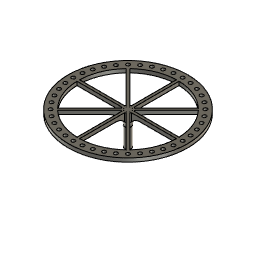
Reaction_Wheel (Autodesk Fusion 360 design; units mm, degrees)
Autodesk Fusion 360 part; units mm, degrees
note: some values were not read from the file. Chosen so that the rebuilt part matches the saved one: which pieces of a blend or face edit are solid.
sketch "스케치1" plane through (0, 0, 0) normal (0, 0, 1) x (1, 0, 0)
  circle A0 centre (0, 0) radius 1.6
  circle A1 centre (0, 0) radius 3.3
  dimension "d1" = 3.2
  dimension "d2" = 6.6
  constraint coincident A0.centre A1.centre
  measures "d1" diameter of A0
  measures "d2" diameter of A1
extrude "돌출1" add sketch "스케치1" along normal blind 30 makes body 1
sketch "스케치2" plane through (0, 0, 30) normal (0, 0, 1) x (-1, 0, 0)
  circle A0 centre (0, 0) radius 60
  circle A1 centre (0, 0) radius 50
  circle A2 centre (0, 0) radius 3.3
  line L0 (1.310929, -3.028443) -> (1.310929, -49.982812)
  line L1 (-1.310929, -3.028443) -> (-1.310929, -49.982812)
  line L2 (3.068399, -1.214465) -> (36.270152, -34.416218)
  line L3 (1.214465, -3.068399) -> (34.416218, -36.270152)
  line L4 (3.028443, 1.310929) -> (49.982812, 1.310929)
  line L5 (3.028443, -1.310929) -> (49.982812, -1.310929)
  line L6 (1.214465, 3.068399) -> (34.416218, 36.270152)
  line L7 (3.068399, 1.214465) -> (36.270152, 34.416218)
  line L8 (-1.310929, 3.028443) -> (-1.310929, 49.982812)
  line L9 (1.310929, 3.028443) -> (1.310929, 49.982812)
  line L10 (-3.068399, 1.214465) -> (-36.270152, 34.416218)
  line L11 (-1.214465, 3.068399) -> (-34.416218, 36.270152)
  line L12 (-3.028443, -1.310929) -> (-49.982812, -1.310929)
  line L13 (-3.028443, 1.310929) -> (-49.982812, 1.310929)
  line L14 (-1.214465, -3.068399) -> (-34.416218, -36.270152)
  line L15 (-3.068399, -1.214465) -> (-36.270152, -34.416218)
  circle A3 centre (0, 0) radius 5
  dimension "d5" = 120
  dimension "d11" = 100
  dimension "d13" = 360
  dimension "d21" = 10
  constraint coincident A0.centre A1.centre
  constraint concentric A1 A3
  measures "d5" diameter of A0
  measures "d11" diameter of A1
  measures "d21" diameter of A3
extrude "돌출3" add sketch "스케치2" along normal blind 2.7 separate body contours A0 | A1 L4 L5 A3 | A1 L6 L7 A3 | A2 L2 L4 L5 L7 A3 | L4 L7 A3 | A1 L2 L3 A3 | L2 L5 A3 | A2 L4 L6 L7 L9 A3 | A2 L0 L2 L3 L5 A3 | A1 L8 L9 A3 | L6 L9 A3 | A2 | A1 L0 L1 A3 | L0 L3 A3 | A2 L6 L8 L9 L11 A3 | A2 L0 L1 L3 L14 A3 | A1 L10 L11 A3 | L8 L11 A3 | A1 L14 L15 A3 | L1 L14 A3 | A2 L8 L10 L11 L13 A3 | A2 L1 L12 L14 L15 A3 | A1 L12 L13 A3 | L10 L13 A3 | L12 L15 A3 | A2 L10 L12 L13 L15 A3 picked at (-0.145674, 56.554182) picked at (19.987758, -0.584166) picked at (24.747837, 24.747837) picked at (3.728779, 1.147432) picked at (4.131776, 1.711438) picked at (24.747837, -24.747837) picked at (4.131776, -1.711438) picked at (2.400607, 3.71707) picked at (2.400607, -3.71707) picked at (0, 34.998727) picked at (1.711438, 4.131776) picked at (-0.428905, -0.986319) picked at (0, -34.998727) picked at (1.711438, -4.131776) picked at (0.93088, 4.325851) picked at (-0.93088, -4.325851) picked at (-24.747837, 24.747837) picked at (-1.711438, 4.131776) picked at (-24.747837, -24.747837) picked at (-1.711438, -4.131776) picked at (-3.71707, 2.400607) picked at (-2.400607, -3.71707) picked at (-34.998727, 0) picked at (-4.131776, 1.711438) picked at (-4.131776, -1.711438) picked at (-4.325851, 0.93088) makes body 2
sketch "스케치3" plane through (0, 0, 32.7) normal (0, 0, 1) x (-1, 0, 0)
  circle A0 centre (-55, 0) radius 1.8
  circle A1 centre (-54.322859, -8.603896) radius 1.8
  circle A2 centre (-52.308108, -16.995935) radius 1.8
  circle A3 centre (-49.005359, -24.969477) radius 1.8
  circle A4 centre (-44.495935, -32.328189) radius 1.8
  circle A5 centre (-38.890873, -38.890873) radius 1.8
  circle A6 centre (-32.328189, -44.495935) radius 1.8
  circle A7 centre (-24.969477, -49.005359) radius 1.8
  circle A8 centre (-16.995935, -52.308108) radius 1.8
  circle A9 centre (-8.603896, -54.322859) radius 1.8
  circle A10 centre (0, -55) radius 1.8
  circle A11 centre (8.603896, -54.322859) radius 1.8
  circle A12 centre (16.995935, -52.308108) radius 1.8
  circle A13 centre (24.969477, -49.005359) radius 1.8
  circle A14 centre (32.328189, -44.495935) radius 1.8
  circle A15 centre (38.890873, -38.890873) radius 1.8
  circle A16 centre (44.495935, -32.328189) radius 1.8
  circle A17 centre (49.005359, -24.969477) radius 1.8
  circle A18 centre (52.308108, -16.995935) radius 1.8
  circle A19 centre (54.322859, -8.603896) radius 1.8
  circle A20 centre (55, 0) radius 1.8
  circle A21 centre (54.322859, 8.603896) radius 1.8
  circle A22 centre (52.308108, 16.995935) radius 1.8
  circle A23 centre (49.005359, 24.969477) radius 1.8
  circle A24 centre (44.495935, 32.328189) radius 1.8
  circle A25 centre (38.890873, 38.890873) radius 1.8
  circle A26 centre (32.328189, 44.495935) radius 1.8
  circle A27 centre (24.969477, 49.005359) radius 1.8
  circle A28 centre (16.995935, 52.308108) radius 1.8
  circle A29 centre (8.603896, 54.322859) radius 1.8
  circle A30 centre (0, 55) radius 1.8
  circle A31 centre (-8.603896, 54.322859) radius 1.8
  circle A32 centre (-16.995935, 52.308108) radius 1.8
  circle A33 centre (-24.969477, 49.005359) radius 1.8
  circle A34 centre (-32.328189, 44.495935) radius 1.8
  circle A35 centre (-38.890873, 38.890873) radius 1.8
  circle A36 centre (-44.495935, 32.328189) radius 1.8
  circle A37 centre (-49.005359, 24.969477) radius 1.8
  circle A38 centre (-52.308108, 16.995935) radius 1.8
  circle A39 centre (-54.322859, 8.603896) radius 1.8
  dimension "d16" = 3.6
  dimension "d18" = 360
  measures "d16" diameter of A0
extrude "돌출4" cut sketch "스케치3" against normal through all bodies 2
extrude "돌출5" add sketch "스케치2" against normal blind 1 contours A1 L4 L5 A3 | A1 L6 L7 A3 | A2 L2 L4 L5 L7 A3 | L4 L7 A3 | A1 L2 L3 A3 | L2 L5 A3 | A2 L4 L6 L7 L9 A3 | A2 L4 L7 | A2 L0 L2 L3 L5 A3 | A2 L2 L5 | A1 L8 L9 A3 | L6 L9 A3 | A1 L0 L1 A3 | L0 L3 A3 | A2 L6 L8 L9 L11 A3 | A2 L6 L9 | A2 L0 L1 L3 L14 A3 | A2 L0 L3 | A1 L10 L11 A3 | L8 L11 A3 | A1 L14 L15 A3 | L1 L14 A3 | A2 L8 L10 L11 L13 A3 | A2 L8 L11 | A2 L1 L12 L14 L15 A3 | A2 L1 L14 | A1 L12 L13 A3 | L10 L13 A3 | L12 L15 A3 | A2 L10 L12 L13 L15 A3 | A2 L10 L13 | A2 L12 L15 picked at (19.987758, -0.584166) picked at (24.747837, 24.747837) picked at (3.728779, 1.147432) picked at (4.131776, 1.711438) picked at (24.747837, -24.747837) picked at (4.131776, -1.711438) picked at (2.400607, 3.71707) picked at (3.087461, 1.278868) picked at (2.400607, -3.71707) picked at (3.087461, -1.278868) picked at (0, 34.998727) picked at (1.711438, 4.131776) picked at (0, -34.998727) picked at (1.711438, -4.131776) picked at (0.93088, 4.325851) picked at (1.278868, 3.087461) picked at (-0.93088, -4.325851) picked at (1.278868, -3.087461) picked at (-24.747837, 24.747837) picked at (-1.711438, 4.131776) picked at (-24.747837, -24.747837) picked at (-1.711438, -4.131776) picked at (-3.71707, 2.400607) picked at (-1.278868, 3.087461) picked at (-2.400607, -3.71707) picked at (-1.278868, -3.087461) picked at (-34.998727, 0) picked at (-4.131776, 1.711438) picked at (-4.131776, -1.711438) picked at (-4.325851, 0.93088) picked at (-3.087461, 1.278868) picked at (-3.087461, -1.278868) bodies 1 2
fillet "모깎기1" radius 10 1 edges at (-3.07668, 1.193331, 29) on bodies 1
extrude "돌출6" add 1 faces at (57.357273, -12.222724, 30) along direction (0, 0, -1) blind 1 on bodies 1 bodies 1
